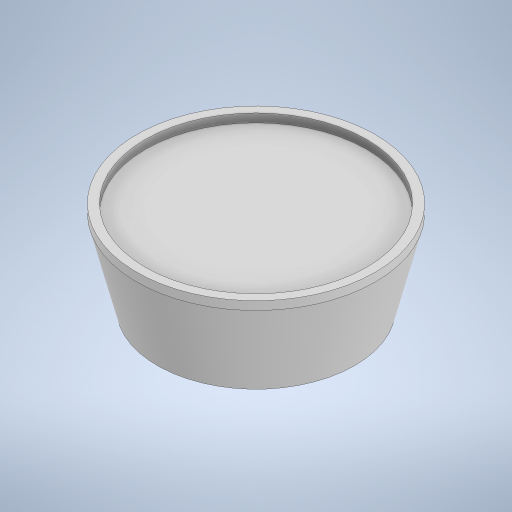
# Autodesk Inventor part: 屋-1 base
Saved by Autodesk Inventor 2024 (Build 280153000, 153)
## iProperties
Created: 2024-05-19
Part Number: 屋-1 base
Material: 一般
Document SubType Name: Modeling
Designer: User
Density: 1 g/cm^3
Appearance: 預設
Author: User
Autodesk Inventor part; units mm, degrees
ref_plane "YZ Plane" through (0, 0, 0) normal (1, 0, 0) x (0, 1, 0)
ref_plane "XZ Plane" through (0, 0, 0) normal (0, 1, 0) x (-1, 0, 0)
ref_plane "XY Plane" through (0, 0, 0) normal (0, 0, 1) x (1, 0, 0)
sketch "草圖2" plane through (0, 0, 0) normal (0, 0, 1) x (1, 0, 0)
  line L0 (0, 0) -> (28, 0)
  line L1 (28, 0) -> (23.1748, -19.4092)
  line L2 (23.1748, -19.4092) -> (0, -19.4092)
  line L3 (0, -19.4092) -> (0, 0)
  line L4 (0, 0) -> (0, -19.4092)
  dimension "d1" = 28
  dimension "d2" = 20
  constraints: 10 end point, 1 collinear, 1 horizontal, 1 parallel, 1 perpendicular
  measures "d1" distance of L0.start L0.end
  measures "d2" distance of L0.end L1.end
revolve "迴轉1" add sketch "草圖2" angle 360 about axis through (0, -19.4092, 0) along (0, 1, 0)
sketch "草圖3" plane through (0, 0, 0) normal (0, 1, 0) x (1, 0, 0)
  circle A0 centre (0, 0) radius 28
  circle A1 centre (0, 0) radius 26
  dimension "d4" = 56
  dimension "d5" = 52
  constraints: 2 centre point, 2 coincident
  measures "d4" diameter of A0
  measures "d5" diameter of A1
extrude "擠出1" add sketch "草圖3" along normal blind 2
